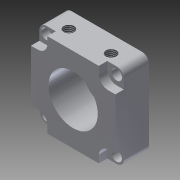
# Autodesk Inventor part: Gearbox End Plate
Saved by Autodesk Inventor 2013 (Build 170138000, 138)
## iProperties
Created: 2012-01-14
Part Number: Gearbox End Plate
Material: Aluminum-6061
Document SubType Name: Modeling
Designer: Moses
Density: 2.71 g/cm^3
Mass: 38.6775 g
Surface Area: 61.6772 cm^2
Volume: 14.2721 cm^3
Author: Moses
Autodesk Inventor part; units mm, degrees
note: some values were not read from the file. Chosen so that the rebuilt part matches the saved one: sketch regions of "Extrusion2".
ref_plane "YZ Plane" through (0, 0, 0) normal (1, 0, 0) x (0, 1, 0)
ref_plane "XZ Plane" through (0, 0, 0) normal (0, 1, 0) x (-1, 0, 0)
ref_plane "XY Plane" through (0, 0, 0) normal (0, 0, 1) x (1, 0, 0)
sketch "Sketch1" plane through (0, 0, 0) normal (0, 0, 1) x (1, 0, 0)
  line L0 (0, 0) -> (38.1, 0)
  line L1 (38.1, 0) -> (38.1, 38.1)
  line L2 (38.1, 38.1) -> (0, 38.1)
  line L3 (0, 38.1) -> (0, 0)
  circle A0 centre (3.175, 34.925) radius 2.3495
  circle A1 centre (34.925, 34.925) radius 2.3495
  circle A2 centre (3.175, 3.175) radius 2.3495
  circle A3 centre (34.925, 3.175) radius 2.3495
  line L4 (0, 19.05) -> (19.05, 19.05)
  circle A4 centre (19.05, 19.05) radius 11.1125
  circle A5 centre (19.05, 19.05) radius 6.35
  line L5 (7.4295, 34.925) -> (7.4295, 38.1)
  line L6 (0, 30.6705) -> (3.175, 30.6705)
  arc A6 (3.175, 30.6705) -> (7.4295, 34.925) centre (3.175, 34.925) ccw
  line L7 (5.5245, 34.925) -> (7.4295, 34.925)
  line L8 (3.175, 7.4295) -> (0, 7.4295)
  line L9 (7.4295, 0) -> (7.4295, 3.175)
  arc A7 (7.4295, 3.175) -> (3.175, 7.4295) centre (3.175, 3.175) ccw
  line L10 (30.6705, 3.175) -> (30.6705, 0)
  line L11 (38.1, 7.4295) -> (34.925, 7.4295)
  arc A8 (34.925, 7.4295) -> (30.6705, 3.175) centre (34.925, 3.175) ccw
  line L12 (34.925, 30.6705) -> (38.1, 30.6705)
  line L13 (30.6705, 38.1) -> (30.6705, 34.925)
  arc A9 (30.6705, 34.925) -> (34.925, 30.6705) centre (34.925, 34.925) ccw
  line L14 (0, 7.4295) -> (0, 0)
  line L15 (0, 0) -> (7.4295, 0)
  line L16 (30.6705, 0) -> (38.1, 0)
  line L17 (38.1, 0) -> (38.1, 7.4295)
  line L18 (30.6705, 38.1) -> (38.1, 38.1)
  line L19 (38.1, 38.1) -> (38.1, 30.6705)
  dimension "d2" = 4.699
  dimension "d0" = 38.1
  dimension "d1" = 38.1
  dimension "d5" = 31.75
  dimension "d8" = 31.75
  dimension "d11" = 3.175
  dimension "d12" = 3.175
  dimension "d13" = 19.05
  dimension "d14" = 22.225
  dimension "d15" = 12.7
  dimension "d16" = 3.175
  dimension "d17" = 3.175
  dimension "d18" = 1.905
  dimension "d24" = 360
  constraints: 40 end point, 9 centre point, 8 point on circle, 5 perpendicular, 3 coincident, 2 horizontal, 2 parallel, 2 point on line, 1 collinear, 1 horizontal alignment, 1 midpoint, 1 vertical, 41 other
  measures "d0" distance of L0.start L0.end
  measures "d1" distance of L0.end L1.end
  measures "d5" distance of point (3.175, 34.925) A1.centre
  measures "d8" distance of point (3.175, 34.925) A2.centre
  measures "d11" distance from line of L2 point (3.175, 34.925)
  measures "d12" distance from line of L3 point (3.175, 34.925)
  measures "d13" distance of L4.start L4.end
  measures "d14" diameter of A4
  measures "d15" diameter of A5
  measures "d16" distance of L5.start L5.end
  measures "d17" distance of L6.start L6.end
  measures "d18" distance of L7.start L5.start
extrude "Extrusion1" add sketch "Sketch1" along normal blind 3.81 contours L9 A7 L8 L3 L6 A6 L5 L2 L13 A9 L12 L1 L11 A8 L10 L0
extrude "Extrusion2" add sketch "Sketch1" against normal blind 11.43 contours L3 L8 A7 L9 L0 | L9 A7 L8 L3 L6 A6 L5 L2 L13 A9 L12 L1 L11 A8 L10 L0 | L10 A8 L11 L1 L0 | L3 L2 L5 A6 L6 | L12 A9 L13 L2 L1
fillet "Fillet1" radius 3.175 4 edges at (38.1, 38.1, -5.715) (38.1, 0, -5.715) (0, 38.1, -5.715) (0, 0, -5.715)
sketch "Sketch2" plane through (7.4295, 38.1, 3.81) normal (0, 1, 0) x (1, 0, 0)
  line L0 (11.6205, 7.62) -> (21.1455, 7.62)
  line L1 (11.6205, 7.62) -> (2.0955, 7.62)
  circle A0 centre (2.0955, 7.62) radius 2.3495
  circle A1 centre (21.1455, 7.62) radius 2.3495
  line L2 (0, 0) -> (23.241, 0) projected
  line L3 (11.6205, 7.62) -> (11.6205, 0)
  point P0 (-7.4295, 3.81)
  dimension "d32" = 9.525
  dimension "d33" = 9.525
  dimension "d34" = 4.699
  dimension "d35" = 4.699
  dimension "d45" = 7.62
  constraints: 6 end point, 2 centre point, 2 coincident, 1 collinear, 1 horizontal, 1 midpoint, 1 vertical
  measures "d32" distance of L0.start L0.end
  measures "d33" distance of L0.start L1.end
  measures "d34" diameter of A0
  measures "d35" diameter of A1
  measures "d45" distance of L0.start L3.end
extrude "Extrusion3" cut sketch "Sketch2" against normal blind 3.81
sketch "Sketch3" plane through (7.4295, 0, 3.81) normal (0, -1, 0) x (1, 0, 0)
  line L0 (11.6205, -7.62) -> (21.1455, -7.62)
  line L1 (11.6205, -7.62) -> (2.0955, -7.62)
  circle A0 centre (2.0955, -7.62) radius 2.3495
  circle A1 centre (21.1455, -7.62) radius 2.3495
  line L2 (23.241, 0) -> (0, 0) projected
  line L3 (11.6205, -7.62) -> (11.6205, 0)
  point P0 (-7.4295, -3.81)
  dimension "d39" = 9.525
  dimension "d40" = 9.525
  dimension "d41" = 4.699
  dimension "d42" = 4.699
  dimension "d46" = 7.62
  constraints: 6 end point, 2 centre point, 2 coincident, 1 collinear, 1 horizontal, 1 midpoint, 1 vertical
  measures "d39" distance of L0.start L0.end
  measures "d40" distance of L0.start L1.end
  measures "d41" diameter of A0
  measures "d42" diameter of A1
  measures "d46" distance of L0.start L3.end
extrude "Extrusion4" cut sketch "Sketch3" against normal blind 3.81
thread "Thread1" size "10-32 UNF" class "2B" standard "ANSI Unified Screw Threads" full length
thread "Thread2" size "10-32 UNF" class "2B" standard "ANSI Unified Screw Threads" full length
thread "Thread3" size "10-32 UNF" class "2B" standard "ANSI Unified Screw Threads" full length
thread "Thread4" size "10-32 UNF" class "2B" standard "ANSI Unified Screw Threads" full length
equation "\"d16\" = d11"
equation "\"d17\" = d11"
body "Solid1"
